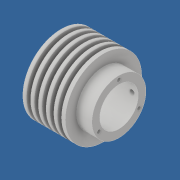
# Autodesk Inventor part: Kühlkörper
Saved by Autodesk Inventor 2018 (Build 220112000, 112)
## iProperties
Created: 2018-10-02
Part Number: Kühlkörper
Material: Generisch
Document SubType Name: Modeling
Designer: M.Knabel
Density: 1 g/cm^3
Appearance: Vorgabe
Author: M.Knabel
Autodesk Inventor part; units mm, degrees
ref_plane "YZ Plane" through (0, 0, 0) normal (1, 0, 0) x (0, 1, 0)
ref_plane "XY Plane" through (0, 0, 0) normal (0, 0, 1) x (1, 0, 0)
sketch "Skizze2" plane through (0, 0, 0) normal (0, 0, 1) x (1, 0, 0)
  line L0 (0, -4.95) -> (0, 29.7) projected
  line L1 (-7.5, 0) -> (45, 0) projected
  line L2 (10, 12.5) -> (37.5, 12.5)
  line L3 (37.5, 12.5) -> (37.5, 17.5)
  line L4 (37.5, 17.5) -> (27.5, 17.5)
  line L5 (27.5, 17.5) -> (27.5, 24.75)
  line L6 (27.5, 24.75) -> (25, 24.75)
  line L7 (25, 24.75) -> (25, 17.5)
  line L8 (25, 17.5) -> (22.4, 17.5)
  line L9 (22.4, 17.5) -> (22.4, 24.75)
  line L10 (22.4, 24.75) -> (20, 24.75)
  line L11 (20, 24.75) -> (20, 17.5)
  line L12 (20, 17.5) -> (17.4, 17.5)
  line L13 (17.4, 17.5) -> (17.4, 24.75)
  line L14 (17.4, 24.75) -> (15, 24.75)
  line L15 (15, 24.75) -> (15, 17.5)
  line L16 (15, 17.5) -> (12.4, 17.5)
  line L17 (12.4, 17.5) -> (12.4, 24.75)
  line L18 (12.4, 24.75) -> (10, 24.75)
  line L19 (10, 24.75) -> (10, 17.5)
  line L20 (10, 17.5) -> (7.4, 17.5)
  line L21 (7.4, 17.5) -> (7.4, 24.75)
  line L22 (7.4, 24.75) -> (5, 24.75)
  line L23 (5, 24.75) -> (5, 17.5)
  line L24 (5, 17.5) -> (2.4, 17.5)
  line L25 (2.4, 17.5) -> (2.4, 24.75)
  line L26 (2.4, 24.75) -> (0, 24.75)
  line L27 (0, 24.75) -> (0, 15)
  line L28 (0, 15) -> (10, 15)
  line L29 (10, 15) -> (10, 12.5)
  point P0 (0, 0)
  dimension "d3" = 37.5
  dimension "d4" = 10
  dimension "d5" = 49.5
  dimension "d6" = 35
  dimension "d7" = 2.4
  dimension "d8" = 2.6
  dimension "d10" = 25
  dimension "d11" = 10
  dimension "d13" = 2.4
  dimension "d14" = 25
  dimension "d15" = 30
  dimension "d16" = 2.4
  dimension "d17" = 2.6
  dimension "d19" = 2.4
  dimension "d20" = 2.6
  dimension "d21" = 2.4
  constraints: 56 end point, 19 point on line, 16 perpendicular, 2 collinear, 1 horizontal, 1 parallel
  measures "d3" distance between parallel lines of L3 L27
  measures "d4" distance between parallel lines of L3 L5
  measures "d5" diameter of L26 L1
  measures "d6" diameter of L24 L1
  measures "d7" distance between parallel lines of L25 L27
  measures "d8" distance between parallel lines of L23 L25
  measures "d10" distance between parallel lines of L7 L27
  measures "d11" distance between parallel lines of L29 L27
  measures "d13" distance between parallel lines of L21 L23
  measures "d14" diameter of L2 L1
  measures "d15" diameter of L28 L1
  measures "d16" distance between parallel lines of L19 L17
  measures "d17" distance between parallel lines of L15 L17
  measures "d19" distance between parallel lines of L13 L15
  measures "d20" distance between parallel lines of L11 L13
  measures "d21" distance between parallel lines of L9 L11
revolve "Umdrehung1" add sketch "Skizze2" angle 360 about axis through (-10, 0, 0) along (1, 0, 0)
sketch "Skizze4" plane through (37.5, 0, 0) normal (1, 0, 0) x (0, 0, -1)
  line L0 (0, -34.65) -> (0, 34.65) projected
  line L1 (34.65, 0) -> (-34.65, 0) projected
  circle A0 centre (0, 0) radius 15 projected
  point P0 (-15, 0)
  constraints: 1 horizontal alignment, 1 point on line, 1 other
hole "Bohrung1" at (37.5, 0, 15) direction (-1, 0, 0) diameter 2.459 depth 8 tip angle 118 thread size "M3x0.5" class "6H" standard "ISO Metric profile"
pattern_circular "Runde Anordnung1" count 3 over 360 about axis through (23.75, 0, 0) along (1, 0, 0) of "Bohrung1"
ref_plane "Arbeitsebene1" through (32.5, 17.5, 0) normal (0, 1, 0) x (-1, 0, 0)
sketch "Skizze5" plane through (32.5, 17.5, 0) normal (0, 1, 0) x (-1, 0, 0)
  line L0 (40, 0) -> (-12.5, 0) projected
  line L1 (-5, 17.5) -> (-5, -17.5) projected
  point P0 (32.5, 0)
  point P1 (-1, 0)
  dimension "d34" = 4
  constraints: 1 point on line
  measures "d34" distance from line of point (-1, 0) L1
hole "Bohrung2" at (33.5, 17.5, 0) direction (0, -1, 0) diameter 3 end up to face face through (23.75, 0, 0) facing (1, 0, 0) round with radius 12.5 far side yes counterbore diameter 4 counterbore depth 3
